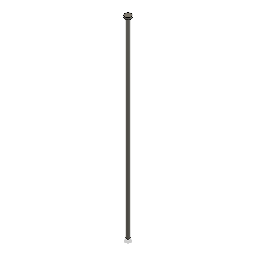
Pepper dryer (Autodesk Fusion 360 archive; units mm, degrees)
design "clou_long"
Autodesk Fusion 360 part; units mm, degrees
sketch "Sketch1" plane through (0, 0, 0) normal (0, 1, 0) x (1, 0, 0)
  circle A0 centre (0, 0) radius 0.5
  dimension "d1" = 1
  measures "d1" diameter of A0
extrude "Extrude1" add sketch "Sketch1" along normal blind 50 makes body 1
extrude "Extrude2" add 1 faces at (0.3557, 50, 0.1033) along direction (0, 1, 0) blind 0.5 separate body on bodies 1 makes body 2
move_face "OffsetFaces1" offset 0.3 1 faces at (0.4975, 50.1667, 0.0498) on bodies 2
chamfer "Chamfer1" distance 0.75 distance2 0.5 1 edges at (-0.4662, 0, 0.1808) measured on face at (-0.3297, 33.3333, -0.3759) on bodies 1
equation "d1 = diamètre"
equation "d2 = longueur"
equation "d4 = hauteur_tête"
equation "d6 = diamètre_tête"
equation "d7 = diamètre * 3 / 4"
equation "d8 = diamètre / 2"
equation "diamètre = 1 mm"
equation "longueur = 50 mm"
equation "épaisseur_tête = 0.2 mm"
equation "diamètre_tête = 0.3 mm"
equation "hauteur_tête = 0.5 mm"
